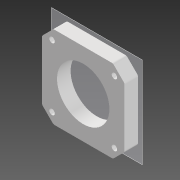
# Autodesk Inventor part: upvulling steppers axis5_6
Saved by Autodesk Inventor 2020 (Build 240168000, 168)
## iProperties
Created: 2020-05-26
Part Number: upvulling steppers axis5_6
Material: ABS Plastic
Document SubType Name: Modeling
Designer: stefa
Density: 1.06 g/cm^3
Appearance: Smooth - Red
Author: stefa
Autodesk Inventor part; units mm, degrees
ref_plane "YZ Plane" through (0, 0, 0) normal (1, 0, 0) x (0, 1, 0)
ref_plane "XZ Plane" through (0, 0, 0) normal (0, 1, 0) x (-1, 0, 0)
ref_plane "XY Plane" through (0, 0, 0) normal (0, 0, 1) x (1, 0, 0)
ref_plane "Work Plane3" through (0, 0, 0) normal (0, 0, 1) x (1, 0, 0)
sketch "Sketch1" plane through (0, 0, 0) normal (0, 0, 1) x (1, 0, 0)
  circle A0 centre (15.5, -15.5) radius 1.25 projected
  circle A1 centre (-15.5, -15.5) radius 1.25 projected
  circle A2 centre (15.5, 15.5) radius 1.25 projected
  circle A3 centre (-15.5, 15.5) radius 1.25 projected
  circle A4 centre (0, 0) radius 11 projected
  line L0 (-14.1716, 20.5) -> (14.1716, 20.5) projected
  arc A5 (-14.1716, 20.5) -> (-15.2322, 20.0607) centre (-14.1716, 19) ccw projected
  line L1 (-20.0607, 15.2322) -> (-15.2322, 20.0607) projected
  arc A6 (-20.0607, 15.2322) -> (-20.5, 14.1716) centre (-19, 14.1716) ccw projected
  line L2 (-20.5, -14.1716) -> (-20.5, 14.1716) projected
  arc A7 (-20.5, -14.1716) -> (-20.0607, -15.2322) centre (-19, -14.1716) ccw projected
  line L3 (-15.2322, -20.0607) -> (-20.0607, -15.2322) projected
  arc A8 (-15.2322, -20.0607) -> (-14.1716, -20.5) centre (-14.1716, -19) ccw projected
  line L4 (14.1716, -20.5) -> (-14.1716, -20.5) projected
  arc A9 (14.1716, -20.5) -> (15.2322, -20.0607) centre (14.1716, -19) ccw projected
  line L5 (20.0607, -15.2322) -> (15.2322, -20.0607) projected
  arc A10 (20.0607, -15.2322) -> (20.5, -14.1716) centre (19, -14.1716) ccw projected
  line L6 (20.5, 14.1716) -> (20.5, -14.1716) projected
  arc A11 (20.5, 14.1716) -> (20.0607, 15.2322) centre (19, 14.1716) ccw projected
  line L7 (15.2322, 20.0607) -> (20.0607, 15.2322) projected
  arc A12 (15.2322, 20.0607) -> (14.1716, 20.5) centre (14.1716, 19) ccw projected
  circle A13 centre (0, 0) radius 13
  circle A14 centre (-15.5, -15.5) radius 1.35
  circle A15 centre (-15.5, 15.5) radius 1.35
  circle A16 centre (15.5, 15.5) radius 1.35
  circle A17 centre (15.5, -15.5) radius 1.35
  point P0 (0, 0)
  dimension "d0" = 2
  dimension "d1" = 0.1
  dimension "d2" = 0.1
  dimension "d3" = 0.1
  dimension "d4" = 0.1
  constraints: 5 centre point
  measures "d0" radial gap between concentric circles of A4 A13
  measures "d1" radial gap between concentric circles of A1 A14
  measures "d2" radial gap between concentric circles of A3 A15
  measures "d3" radial gap between concentric circles of A2 A16
  measures "d4" radial gap between concentric circles of A0 A17
extrude "Extrusion1" add sketch "Sketch1" along normal blind 6.75 contours L0 A12 L7 A11 L6 A10 L5 A9 L4 A8 L3 A7 L2 A6 L1 A5
body "Solid1"
